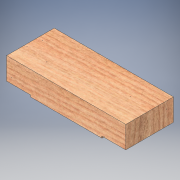
# Autodesk Inventor part: lifterBase
Saved by Autodesk Inventor 2017 (Build 210142000, 142)
## iProperties
Created: 2017-02-02
Part Number: lifterBase
Material: Generic
Document SubType Name: Modeling
Designer: kingb
Density: 1 g/cm^3
Appearance: Birch - Natural Polished
Author: kingb
Autodesk Inventor part; units mm, degrees
ref_plane "YZ Plane" through (0, 0, 0) normal (1, 0, 0) x (0, 1, 0)
ref_plane "XZ Plane" through (0, 0, 0) normal (0, 1, 0) x (-1, 0, 0)
ref_plane "XY Plane" through (0, 0, 0) normal (0, 0, 1) x (1, 0, 0)
sketch "Sketch1" plane through (0, 0, 0) normal (1, 0, 0) x (0, 1, 0)
  line L0 (0, 0) -> (50.8, 0)
  line L1 (50.8, 0) -> (50.8, -101.6)
  line L2 (50.8, -101.6) -> (0, -101.6)
  line L3 (0, -101.6) -> (0, 0)
  dimension "d0" = 50.8
  dimension "d1" = 101.6
  constraints: 8 end point, 2 parallel, 1 horizontal, 1 perpendicular
  measures "d0" distance of L1.end L2.end
  measures "d1" distance of L0.end L1.end
extrude "Extrusion1" add sketch "Sketch1" along normal blind 254
sketch "Sketch2" plane through (0, 0, 0) normal (0, 0, 1) x (1, 0, 0)
  line L0 (0, 0) -> (0, 50.8) projected
  line L1 (0, 0) -> (254, 0) projected
  line L2 (254, 50.8) -> (254, 0) projected
  line L3 (0, 50.8) -> (254, 50.8) projected
  line L4 (0, 0) -> (254, 0) projected
  line L5 (50.8, 0) -> (50.8, 3.81)
  line L6 (50.8, 3.81) -> (0, 3.81)
  line L7 (0, 0) -> (0, 50.8) projected
  line L8 (127, 0) -> (127, 50.8) construction
  line L9 (203.2, 0) -> (203.2, 3.81)
  line L10 (203.2, 3.81) -> (254, 3.81)
  line L11 (50.8, 0) -> (0, 0)
  line L12 (203.2, 0) -> (254, 0)
  line L13 (254, 50.8) -> (254, 0) projected
  line L14 (254, 3.81) -> (254, 0)
  dimension "d4" = 3.81
  dimension "d5" = 90
  dimension "d6" = 50.8
  constraints: 16 end point, 3 symmetric about line, 2 collinear, 2 midpoint, 2 point on line, 2 vertical, 1 perpendicular
  measures "d4" distance from line of L1 L5.end
  measures "d5" angle of L1 L5
  measures "d6" distance of L4.start L5.start
extrude "Extrusion2" cut sketch "Sketch2" against normal up to next contours L0 L6 L5 L1 | L9 L10 L2 L1
body "Solid1"
